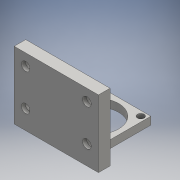
# Autodesk Inventor part: NEMA14 Mounting Bracket
Saved by Autodesk Inventor 2016 (Build 200138000, 138)
## iProperties
Created: 2017-03-15
Part Number: NEMA14 Mounting Bracket
Material: Generic
Document SubType Name: Modeling
Designer: Billy
Density: 1 g/cm^3
Appearance: Default
Author: Billy
Autodesk Inventor part; units mm, degrees
ref_plane "YZ Plane" through (0, 0, 0) normal (1, 0, 0) x (0, 1, 0)
ref_plane "XZ Plane" through (0, 0, 0) normal (0, 1, 0) x (-1, 0, 0)
ref_plane "XY Plane" through (0, 0, 0) normal (0, 0, 1) x (1, 0, 0)
sketch "Sketch1" plane through (0, 0, 0) normal (0, 1, 0) x (-1, 0, 0)
  circle A0 centre (15.9, 35) radius 2.25
  circle A1 centre (15.9, 16) radius 2.25
  circle A2 centre (-15.9, 16) radius 2.25
  circle A3 centre (-15.9, 35) radius 2.25
  line L0 (21.9, 10) -> (-21.9, 10)
  line L1 (-21.9, 10) -> (-21.9, 41)
  line L2 (-21.9, 41) -> (21.9, 41)
  line L3 (21.9, 41) -> (21.9, 10)
  point P0 (0, 0)
  point P1 (0, 0)
  dimension "d0" = 43.8
  dimension "d1" = 31
  constraints: 8 end point, 4 centre point, 2 parallel, 1 horizontal, 1 perpendicular
  measures "d0" distance of L1.end L2.end
  measures "d1" distance of L0.end L1.end
extrude "Extrusion1" add sketch "Sketch1" along normal blind 6
sketch "Sketch2" plane through (0, 6, 0) normal (0, 1, 0) x (1, 0, 0)
  circle A0 centre (-15.9, -16) radius 2.25 projected
  circle A1 centre (-15.9, -16) radius 4
  circle A2 centre (-15.9, -35) radius 2.25 projected
  circle A3 centre (-15.9, -35) radius 4
  circle A4 centre (15.9, -35) radius 2.25 projected
  circle A5 centre (15.9, -35) radius 4
  circle A6 centre (15.9, -16) radius 2.25 projected
  circle A7 centre (15.9, -16) radius 4
  point P0 (0, 0)
  dimension "d4" = 8
  dimension "d5" = 8
  dimension "d6" = 8
  dimension "d7" = 8
  constraints: 4 centre point, 4 coincident
  measures "d4" diameter of A1
  measures "d5" diameter of A3
  measures "d6" diameter of A5
  measures "d7" diameter of A7
extrude "Extrusion2" cut sketch "Sketch2" against normal blind 4
sketch "Sketch4" plane through (21.9, 0, 10) normal (0, 0, -1) x (-1, 0, 0)
  line L0 (43.8, 0) -> (0, 0) projected
  line L1 (43.8, 0) -> (43.8, 6) projected
  line L2 (0, 6) -> (43.8, 6) projected
  line L3 (0, 0) -> (0, 6) projected
  line L4 (0, 6) -> (43.8, 6) projected
  line L5 (36, 6) -> (36, 35)
  line L6 (36, 35) -> (21.9, 35)
  line L7 (36, 35) -> (7.8, 35)
  line L8 (7.8, 35) -> (7.8, 6)
  line L9 (36, 6.8) -> (36, 35)
  line L10 (33.4, 32.4) -> (21.9, 32.4)
  line L11 (10.4, 9.4) -> (33.4, 9.4)
  circle A0 centre (33.4, 32.4) radius 1.75
  circle A1 centre (10.4, 32.4) radius 1.75
  circle A2 centre (10.4, 9.4) radius 1.75
  circle A3 centre (33.4, 9.4) radius 1.75
  circle A4 centre (21.9, 20.9) radius 11.5
  point P0 (21.9, 0)
  dimension "d31" = 14.1
  dimension "d34" = 11.5
  dimension "d39" = 3.5
  dimension "d40" = 3.5
  dimension "d41" = 3.5
  dimension "d42" = 3.5
  dimension "d43" = 23
  constraints: 14 end point, 5 centre point, 3 coincident, 2 point on line, 1 horizontal, 1 parallel, 1 perpendicular
  measures "d31" distance of L6.end L5.end
  measures "d34" distance of L10.end L10.start
  measures "d39" diameter of A0
  measures "d40" diameter of A1
  measures "d41" diameter of A2
  measures "d42" diameter of A3
  measures "d43" diameter of A4
extrude "Extrusion4" add sketch "Sketch4" along normal blind 4
chamfer "Chamfer3" distance 7.8 angle 45 1 edges at (14.1, 6, 8)
chamfer "Chamfer4" distance 7.8 angle 45 1 edges at (-14.1, 6, 8)
body "Solid1"
